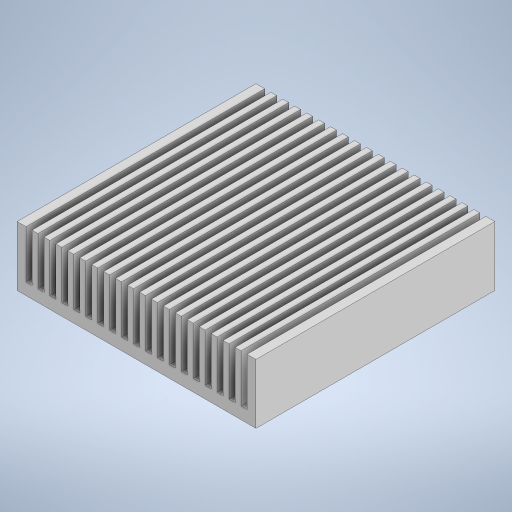
# Autodesk Inventor part: cooling_fin
Saved by Autodesk Inventor 2023 (Build 270158000, 158)
## iProperties
Created: 2023-07-12
Part Number: cooling_fin
Material: 一般
Document SubType Name: Modeling
Designer: 310611102
Density: 1 g/cm^3
Appearance: 預設
Author: 310611102
Autodesk Inventor part; units mm, degrees
ref_plane "YZ Plane" through (0, 0, 0) normal (1, 0, 0) x (0, 1, 0)
ref_plane "XZ Plane" through (0, 0, 0) normal (0, 1, 0) x (-1, 0, 0)
ref_plane "XY Plane" through (0, 0, 0) normal (0, 0, 1) x (1, 0, 0)
sketch "Sketch1" plane through (0, 0, 0) normal (0, 0, 1) x (1, 0, 0)
  line L0 (-10, 2.5) -> (10, 2.5)
  line L1 (10, 2.5) -> (10, -2.5)
  line L2 (10, -2.5) -> (-10, -2.5)
  line L3 (-10, -2.5) -> (-10, 2.5)
  line L4 (-10, 2.5) -> (10, -2.5) construction
  line L5 (10, 2.5) -> (-10, -2.5) construction
  point P0 (0, 0)
  dimension "d0" = 20
  dimension "d1" = 5
  constraints: 12 end point, 2 midpoint, 2 parallel, 1 horizontal, 1 perpendicular
  measures "d0" distance of L0.start L0.end
  measures "d1" distance of L0.end L1.end
extrude "Extrusion1" add sketch "Sketch1" along normal blind 20
sketch "Sketch2" plane through (0, 0, 20) normal (0, 0, 1) x (1, 0, 0)
  line L0 (-0.25, 3.3824) -> (0.25, 3.3824)
  line L1 (0.25, 3.3824) -> (0.25, -1.5)
  line L2 (0.25, -1.5) -> (-0.25, -1.5)
  line L3 (-0.25, -1.5) -> (-0.25, 3.3824)
  line L4 (-0.25, 3.3824) -> (0.25, -1.5) construction
  line L5 (0.25, 3.3824) -> (-0.25, -1.5) construction
  line L6 (-10, -2.5) -> (10, -2.5) projected
  line L7 (0.75, 3.3824) -> (1.25, 3.3824)
  line L8 (1.25, 3.3824) -> (1.25, -1.5)
  line L9 (1.25, -1.5) -> (0.75, -1.5)
  line L10 (0.75, -1.5) -> (0.75, 3.3824)
  line L11 (0.75, 3.3824) -> (1.25, -1.5) construction
  line L12 (1.25, 3.3824) -> (0.75, -1.5) construction
  line L13 (1.75, 3.3824) -> (2.25, 3.3824)
  line L14 (2.25, 3.3824) -> (2.25, -1.5)
  line L15 (2.25, -1.5) -> (1.75, -1.5)
  line L16 (1.75, -1.5) -> (1.75, 3.3824)
  line L17 (1.75, 3.3824) -> (2.25, -1.5) construction
  line L18 (2.25, 3.3824) -> (1.75, -1.5) construction
  line L19 (2.75, 3.3824) -> (3.25, 3.3824)
  line L20 (3.25, 3.3824) -> (3.25, -1.5)
  line L21 (3.25, -1.5) -> (2.75, -1.5)
  line L22 (2.75, -1.5) -> (2.75, 3.3824)
  line L23 (2.75, 3.3824) -> (3.25, -1.5) construction
  line L24 (3.25, 3.3824) -> (2.75, -1.5) construction
  line L25 (3.75, 3.3824) -> (4.25, 3.3824)
  line L26 (4.25, 3.3824) -> (4.25, -1.5)
  line L27 (4.25, -1.5) -> (3.75, -1.5)
  line L28 (3.75, -1.5) -> (3.75, 3.3824)
  line L29 (3.75, 3.3824) -> (4.25, -1.5) construction
  line L30 (4.25, 3.3824) -> (3.75, -1.5) construction
  line L31 (4.75, 3.3824) -> (5.25, 3.3824)
  line L32 (5.25, 3.3824) -> (5.25, -1.5)
  line L33 (5.25, -1.5) -> (4.75, -1.5)
  line L34 (4.75, -1.5) -> (4.75, 3.3824)
  line L35 (4.75, 3.3824) -> (5.25, -1.5) construction
  line L36 (5.25, 3.3824) -> (4.75, -1.5) construction
  line L37 (5.75, 3.3824) -> (6.25, 3.3824)
  line L38 (6.25, 3.3824) -> (6.25, -1.5)
  line L39 (6.25, -1.5) -> (5.75, -1.5)
  line L40 (5.75, -1.5) -> (5.75, 3.3824)
  line L41 (5.75, 3.3824) -> (6.25, -1.5) construction
  line L42 (6.25, 3.3824) -> (5.75, -1.5) construction
  line L43 (6.75, 3.3824) -> (7.25, 3.3824)
  line L44 (7.25, 3.3824) -> (7.25, -1.5)
  line L45 (7.25, -1.5) -> (6.75, -1.5)
  line L46 (6.75, -1.5) -> (6.75, 3.3824)
  line L47 (6.75, 3.3824) -> (7.25, -1.5) construction
  line L48 (7.25, 3.3824) -> (6.75, -1.5) construction
  line L49 (7.75, 3.3824) -> (8.25, 3.3824)
  line L50 (8.25, 3.3824) -> (8.25, -1.5)
  line L51 (8.25, -1.5) -> (7.75, -1.5)
  line L52 (7.75, -1.5) -> (7.75, 3.3824)
  line L53 (7.75, 3.3824) -> (8.25, -1.5) construction
  line L54 (8.25, 3.3824) -> (7.75, -1.5) construction
  line L55 (8.75, 3.3824) -> (9.25, 3.3824)
  line L56 (9.25, 3.3824) -> (9.25, -1.5)
  line L57 (9.25, -1.5) -> (8.75, -1.5)
  line L58 (8.75, -1.5) -> (8.75, 3.3824)
  line L59 (8.75, 3.3824) -> (9.25, -1.5) construction
  line L60 (9.25, 3.3824) -> (8.75, -1.5) construction
  line L61 (-1.25, 3.3824) -> (-0.75, 3.3824)
  line L62 (-0.75, 3.3824) -> (-0.75, -1.5)
  line L63 (-0.75, -1.5) -> (-1.25, -1.5)
  line L64 (-1.25, -1.5) -> (-1.25, 3.3824)
  line L65 (-1.25, 3.3824) -> (-0.75, -1.5) construction
  line L66 (-0.75, 3.3824) -> (-1.25, -1.5) construction
  line L67 (-0.25, 3.3824) -> (0.25, 3.3824)
  line L68 (0.25, 3.3824) -> (0.25, -1.5)
  line L69 (0.25, -1.5) -> (-0.25, -1.5)
  line L70 (-0.25, -1.5) -> (-0.25, 3.3824)
  line L71 (-0.25, 3.3824) -> (0.25, -1.5) construction
  line L72 (0.25, 3.3824) -> (-0.25, -1.5) construction
  line L73 (0.75, 3.3824) -> (1.25, 3.3824)
  line L74 (1.25, 3.3824) -> (1.25, -1.5)
  line L75 (1.25, -1.5) -> (0.75, -1.5)
  line L76 (0.75, -1.5) -> (0.75, 3.3824)
  line L77 (0.75, 3.3824) -> (1.25, -1.5) construction
  line L78 (1.25, 3.3824) -> (0.75, -1.5) construction
  line L79 (1.75, 3.3824) -> (2.25, 3.3824)
  line L80 (2.25, 3.3824) -> (2.25, -1.5)
  line L81 (2.25, -1.5) -> (1.75, -1.5)
  line L82 (1.75, -1.5) -> (1.75, 3.3824)
  line L83 (1.75, 3.3824) -> (2.25, -1.5) construction
  line L84 (2.25, 3.3824) -> (1.75, -1.5) construction
  line L85 (2.75, 3.3824) -> (3.25, 3.3824)
  line L86 (3.25, 3.3824) -> (3.25, -1.5)
  line L87 (3.25, -1.5) -> (2.75, -1.5)
  line L88 (2.75, -1.5) -> (2.75, 3.3824)
  line L89 (2.75, 3.3824) -> (3.25, -1.5) construction
  line L90 (3.25, 3.3824) -> (2.75, -1.5) construction
  line L91 (3.75, 3.3824) -> (4.25, 3.3824)
  line L92 (4.25, 3.3824) -> (4.25, -1.5)
  line L93 (4.25, -1.5) -> (3.75, -1.5)
  line L94 (3.75, -1.5) -> (3.75, 3.3824)
  line L95 (3.75, 3.3824) -> (4.25, -1.5) construction
  line L96 (4.25, 3.3824) -> (3.75, -1.5) construction
  line L97 (4.75, 3.3824) -> (5.25, 3.3824)
  line L98 (5.25, 3.3824) -> (5.25, -1.5)
  line L99 (5.25, -1.5) -> (4.75, -1.5)
  line L100 (4.75, -1.5) -> (4.75, 3.3824)
  line L101 (4.75, 3.3824) -> (5.25, -1.5) construction
  line L102 (5.25, 3.3824) -> (4.75, -1.5) construction
  line L103 (5.75, 3.3824) -> (6.25, 3.3824)
  line L104 (6.25, 3.3824) -> (6.25, -1.5)
  line L105 (6.25, -1.5) -> (5.75, -1.5)
  line L106 (5.75, -1.5) -> (5.75, 3.3824)
  line L107 (5.75, 3.3824) -> (6.25, -1.5) construction
  line L108 (6.25, 3.3824) -> (5.75, -1.5) construction
  line L109 (6.75, 3.3824) -> (7.25, 3.3824)
  line L110 (7.25, 3.3824) -> (7.25, -1.5)
  line L111 (7.25, -1.5) -> (6.75, -1.5)
  line L112 (6.75, -1.5) -> (6.75, 3.3824)
  line L113 (6.75, 3.3824) -> (7.25, -1.5) construction
  line L114 (7.25, 3.3824) -> (6.75, -1.5) construction
  line L115 (7.75, 3.3824) -> (8.25, 3.3824)
  line L116 (8.25, 3.3824) -> (8.25, -1.5)
  line L117 (8.25, -1.5) -> (7.75, -1.5)
  line L118 (7.75, -1.5) -> (7.75, 3.3824)
  line L119 (7.75, 3.3824) -> (8.25, -1.5) construction
  line L120 (8.25, 3.3824) -> (7.75, -1.5) construction
  line L121 (-2.25, 3.3824) -> (-1.75, 3.3824)
  line L122 (-1.75, 3.3824) -> (-1.75, -1.5)
  line L123 (-1.75, -1.5) -> (-2.25, -1.5)
  line L124 (-2.25, -1.5) -> (-2.25, 3.3824)
  line L125 (-2.25, 3.3824) -> (-1.75, -1.5) construction
  line L126 (-1.75, 3.3824) -> (-2.25, -1.5) construction
  line L127 (-1.25, 3.3824) -> (-0.75, 3.3824)
  line L128 (-0.75, 3.3824) -> (-0.75, -1.5)
  line L129 (-0.75, -1.5) -> (-1.25, -1.5)
  line L130 (-1.25, -1.5) -> (-1.25, 3.3824)
  line L131 (-1.25, 3.3824) -> (-0.75, -1.5) construction
  line L132 (-0.75, 3.3824) -> (-1.25, -1.5) construction
  line L133 (-0.25, 3.3824) -> (0.25, 3.3824)
  line L134 (0.25, 3.3824) -> (0.25, -1.5)
  line L135 (0.25, -1.5) -> (-0.25, -1.5)
  line L136 (-0.25, -1.5) -> (-0.25, 3.3824)
  line L137 (-0.25, 3.3824) -> (0.25, -1.5) construction
  line L138 (0.25, 3.3824) -> (-0.25, -1.5) construction
  line L139 (0.75, 3.3824) -> (1.25, 3.3824)
  line L140 (1.25, 3.3824) -> (1.25, -1.5)
  line L141 (1.25, -1.5) -> (0.75, -1.5)
  line L142 (0.75, -1.5) -> (0.75, 3.3824)
  line L143 (0.75, 3.3824) -> (1.25, -1.5) construction
  line L144 (1.25, 3.3824) -> (0.75, -1.5) construction
  line L145 (1.75, 3.3824) -> (2.25, 3.3824)
  line L146 (2.25, 3.3824) -> (2.25, -1.5)
  line L147 (2.25, -1.5) -> (1.75, -1.5)
  line L148 (1.75, -1.5) -> (1.75, 3.3824)
  line L149 (1.75, 3.3824) -> (2.25, -1.5) construction
  line L150 (2.25, 3.3824) -> (1.75, -1.5) construction
  line L151 (2.75, 3.3824) -> (3.25, 3.3824)
  line L152 (3.25, 3.3824) -> (3.25, -1.5)
  line L153 (3.25, -1.5) -> (2.75, -1.5)
  line L154 (2.75, -1.5) -> (2.75, 3.3824)
  line L155 (2.75, 3.3824) -> (3.25, -1.5) construction
  line L156 (3.25, 3.3824) -> (2.75, -1.5) construction
  line L157 (3.75, 3.3824) -> (4.25, 3.3824)
  line L158 (4.25, 3.3824) -> (4.25, -1.5)
  line L159 (4.25, -1.5) -> (3.75, -1.5)
  line L160 (3.75, -1.5) -> (3.75, 3.3824)
  line L161 (3.75, 3.3824) -> (4.25, -1.5) construction
  line L162 (4.25, 3.3824) -> (3.75, -1.5) construction
  line L163 (4.75, 3.3824) -> (5.25, 3.3824)
  line L164 (5.25, 3.3824) -> (5.25, -1.5)
  line L165 (5.25, -1.5) -> (4.75, -1.5)
  line L166 (4.75, -1.5) -> (4.75, 3.3824)
  line L167 (4.75, 3.3824) -> (5.25, -1.5) construction
  line L168 (5.25, 3.3824) -> (4.75, -1.5) construction
  line L169 (5.75, 3.3824) -> (6.25, 3.3824)
  line L170 (6.25, 3.3824) -> (6.25, -1.5)
  line L171 (6.25, -1.5) -> (5.75, -1.5)
  line L172 (5.75, -1.5) -> (5.75, 3.3824)
  line L173 (5.75, 3.3824) -> (6.25, -1.5) construction
  line L174 (6.25, 3.3824) -> (5.75, -1.5) construction
  line L175 (6.75, 3.3824) -> (7.25, 3.3824)
  line L176 (7.25, 3.3824) -> (7.25, -1.5)
  line L177 (7.25, -1.5) -> (6.75, -1.5)
  line L178 (6.75, -1.5) -> (6.75, 3.3824)
  line L179 (6.75, 3.3824) -> (7.25, -1.5) construction
  line L180 (7.25, 3.3824) -> (6.75, -1.5) construction
  line L181 (-3.25, 3.3824) -> (-2.75, 3.3824)
  line L182 (-2.75, 3.3824) -> (-2.75, -1.5)
  line L183 (-2.75, -1.5) -> (-3.25, -1.5)
  line L184 (-3.25, -1.5) -> (-3.25, 3.3824)
  line L185 (-3.25, 3.3824) -> (-2.75, -1.5) construction
  line L186 (-2.75, 3.3824) -> (-3.25, -1.5) construction
  line L187 (-2.25, 3.3824) -> (-1.75, 3.3824)
  line L188 (-1.75, 3.3824) -> (-1.75, -1.5)
  line L189 (-1.75, -1.5) -> (-2.25, -1.5)
  line L190 (-2.25, -1.5) -> (-2.25, 3.3824)
  line L191 (-2.25, 3.3824) -> (-1.75, -1.5) construction
  line L192 (-1.75, 3.3824) -> (-2.25, -1.5) construction
  line L193 (-1.25, 3.3824) -> (-0.75, 3.3824)
  line L194 (-0.75, 3.3824) -> (-0.75, -1.5)
  line L195 (-0.75, -1.5) -> (-1.25, -1.5)
  line L196 (-1.25, -1.5) -> (-1.25, 3.3824)
  line L197 (-1.25, 3.3824) -> (-0.75, -1.5) construction
  line L198 (-0.75, 3.3824) -> (-1.25, -1.5) construction
  line L199 (-0.25, 3.3824) -> (0.25, 3.3824)
  line L200 (0.25, 3.3824) -> (0.25, -1.5)
  line L201 (0.25, -1.5) -> (-0.25, -1.5)
  line L202 (-0.25, -1.5) -> (-0.25, 3.3824)
  line L203 (-0.25, 3.3824) -> (0.25, -1.5) construction
  line L204 (0.25, 3.3824) -> (-0.25, -1.5) construction
  line L205 (0.75, 3.3824) -> (1.25, 3.3824)
  line L206 (1.25, 3.3824) -> (1.25, -1.5)
  line L207 (1.25, -1.5) -> (0.75, -1.5)
  line L208 (0.75, -1.5) -> (0.75, 3.3824)
  line L209 (0.75, 3.3824) -> (1.25, -1.5) construction
  line L210 (1.25, 3.3824) -> (0.75, -1.5) construction
  line L211 (1.75, 3.3824) -> (2.25, 3.3824)
  line L212 (2.25, 3.3824) -> (2.25, -1.5)
  line L213 (2.25, -1.5) -> (1.75, -1.5)
  line L214 (1.75, -1.5) -> (1.75, 3.3824)
  line L215 (1.75, 3.3824) -> (2.25, -1.5) construction
  line L216 (2.25, 3.3824) -> (1.75, -1.5) construction
  line L217 (2.75, 3.3824) -> (3.25, 3.3824)
  line L218 (3.25, 3.3824) -> (3.25, -1.5)
  line L219 (3.25, -1.5) -> (2.75, -1.5)
  line L220 (2.75, -1.5) -> (2.75, 3.3824)
  line L221 (2.75, 3.3824) -> (3.25, -1.5) construction
  line L222 (3.25, 3.3824) -> (2.75, -1.5) construction
  line L223 (3.75, 3.3824) -> (4.25, 3.3824)
  line L224 (4.25, 3.3824) -> (4.25, -1.5)
  line L225 (4.25, -1.5) -> (3.75, -1.5)
  line L226 (3.75, -1.5) -> (3.75, 3.3824)
  line L227 (3.75, 3.3824) -> (4.25, -1.5) construction
  line L228 (4.25, 3.3824) -> (3.75, -1.5) construction
  line L229 (4.75, 3.3824) -> (5.25, 3.3824)
  line L230 (5.25, 3.3824) -> (5.25, -1.5)
  line L231 (5.25, -1.5) -> (4.75, -1.5)
  line L232 (4.75, -1.5) -> (4.75, 3.3824)
  line L233 (4.75, 3.3824) -> (5.25, -1.5) construction
  line L234 (5.25, 3.3824) -> (4.75, -1.5) construction
  line L235 (5.75, 3.3824) -> (6.25, 3.3824)
  line L236 (6.25, 3.3824) -> (6.25, -1.5)
  line L237 (6.25, -1.5) -> (5.75, -1.5)
  line L238 (5.75, -1.5) -> (5.75, 3.3824)
  line L239 (5.75, 3.3824) -> (6.25, -1.5) construction
  line L240 (6.25, 3.3824) -> (5.75, -1.5) construction
  line L241 (-4.25, 3.3824) -> (-3.75, 3.3824)
  line L242 (-3.75, 3.3824) -> (-3.75, -1.5)
  line L243 (-3.75, -1.5) -> (-4.25, -1.5)
  line L244 (-4.25, -1.5) -> (-4.25, 3.3824)
  line L245 (-4.25, 3.3824) -> (-3.75, -1.5) construction
  line L246 (-3.75, 3.3824) -> (-4.25, -1.5) construction
  line L247 (-3.25, 3.3824) -> (-2.75, 3.3824)
  line L248 (-2.75, 3.3824) -> (-2.75, -1.5)
  line L249 (-2.75, -1.5) -> (-3.25, -1.5)
  line L250 (-3.25, -1.5) -> (-3.25, 3.3824)
  line L251 (-3.25, 3.3824) -> (-2.75, -1.5) construction
  line L252 (-2.75, 3.3824) -> (-3.25, -1.5) construction
  line L253 (-2.25, 3.3824) -> (-1.75, 3.3824)
  line L254 (-1.75, 3.3824) -> (-1.75, -1.5)
  line L255 (-1.75, -1.5) -> (-2.25, -1.5)
  line L256 (-2.25, -1.5) -> (-2.25, 3.3824)
  line L257 (-2.25, 3.3824) -> (-1.75, -1.5) construction
  line L258 (-1.75, 3.3824) -> (-2.25, -1.5) construction
  line L259 (-1.25, 3.3824) -> (-0.75, 3.3824)
  line L260 (-0.75, 3.3824) -> (-0.75, -1.5)
  line L261 (-0.75, -1.5) -> (-1.25, -1.5)
  line L262 (-1.25, -1.5) -> (-1.25, 3.3824)
  line L263 (-1.25, 3.3824) -> (-0.75, -1.5) construction
  line L264 (-0.75, 3.3824) -> (-1.25, -1.5) construction
  line L265 (-0.25, 3.3824) -> (0.25, 3.3824)
  line L266 (0.25, 3.3824) -> (0.25, -1.5)
  line L267 (0.25, -1.5) -> (-0.25, -1.5)
  line L268 (-0.25, -1.5) -> (-0.25, 3.3824)
  line L269 (-0.25, 3.3824) -> (0.25, -1.5) construction
  line L270 (0.25, 3.3824) -> (-0.25, -1.5) construction
  line L271 (0.75, 3.3824) -> (1.25, 3.3824)
  line L272 (1.25, 3.3824) -> (1.25, -1.5)
  line L273 (1.25, -1.5) -> (0.75, -1.5)
  line L274 (0.75, -1.5) -> (0.75, 3.3824)
  line L275 (0.75, 3.3824) -> (1.25, -1.5) construction
  line L276 (1.25, 3.3824) -> (0.75, -1.5) construction
  line L277 (1.75, 3.3824) -> (2.25, 3.3824)
  line L278 (2.25, 3.3824) -> (2.25, -1.5)
  line L279 (2.25, -1.5) -> (1.75, -1.5)
  line L280 (1.75, -1.5) -> (1.75, 3.3824)
  line L281 (1.75, 3.3824) -> (2.25, -1.5) construction
  line L282 (2.25, 3.3824) -> (1.75, -1.5) construction
  line L283 (2.75, 3.3824) -> (3.25, 3.3824)
  line L284 (3.25, 3.3824) -> (3.25, -1.5)
  line L285 (3.25, -1.5) -> (2.75, -1.5)
  line L286 (2.75, -1.5) -> (2.75, 3.3824)
  line L287 (2.75, 3.3824) -> (3.25, -1.5) construction
  line L288 (3.25, 3.3824) -> (2.75, -1.5) construction
  line L289 (3.75, 3.3824) -> (4.25, 3.3824)
  line L290 (4.25, 3.3824) -> (4.25, -1.5)
  line L291 (4.25, -1.5) -> (3.75, -1.5)
  line L292 (3.75, -1.5) -> (3.75, 3.3824)
  line L293 (3.75, 3.3824) -> (4.25, -1.5) construction
  line L294 (4.25, 3.3824) -> (3.75, -1.5) construction
  line L295 (4.75, 3.3824) -> (5.25, 3.3824)
  line L296 (5.25, 3.3824) -> (5.25, -1.5)
  line L297 (5.25, -1.5) -> (4.75, -1.5)
  line L298 (4.75, -1.5) -> (4.75, 3.3824)
  line L299 (4.75, 3.3824) -> (5.25, -1.5) construction
  line L300 (5.25, 3.3824) -> (4.75, -1.5) construction
  line L301 (-5.25, 3.3824) -> (-4.75, 3.3824)
  line L302 (-4.75, 3.3824) -> (-4.75, -1.5)
  line L303 (-4.75, -1.5) -> (-5.25, -1.5)
  line L304 (-5.25, -1.5) -> (-5.25, 3.3824)
  line L305 (-5.25, 3.3824) -> (-4.75, -1.5) construction
  line L306 (-4.75, 3.3824) -> (-5.25, -1.5) construction
  line L307 (-4.25, 3.3824) -> (-3.75, 3.3824)
  line L308 (-3.75, 3.3824) -> (-3.75, -1.5)
  line L309 (-3.75, -1.5) -> (-4.25, -1.5)
  line L310 (-4.25, -1.5) -> (-4.25, 3.3824)
  line L311 (-4.25, 3.3824) -> (-3.75, -1.5) construction
  line L312 (-3.75, 3.3824) -> (-4.25, -1.5) construction
  line L313 (-3.25, 3.3824) -> (-2.75, 3.3824)
  line L314 (-2.75, 3.3824) -> (-2.75, -1.5)
  line L315 (-2.75, -1.5) -> (-3.25, -1.5)
  line L316 (-3.25, -1.5) -> (-3.25, 3.3824)
  line L317 (-3.25, 3.3824) -> (-2.75, -1.5) construction
  line L318 (-2.75, 3.3824) -> (-3.25, -1.5) construction
  line L319 (-2.25, 3.3824) -> (-1.75, 3.3824)
  line L320 (-1.75, 3.3824) -> (-1.75, -1.5)
  line L321 (-1.75, -1.5) -> (-2.25, -1.5)
  line L322 (-2.25, -1.5) -> (-2.25, 3.3824)
  line L323 (-2.25, 3.3824) -> (-1.75, -1.5) construction
  line L324 (-1.75, 3.3824) -> (-2.25, -1.5) construction
  line L325 (-1.25, 3.3824) -> (-0.75, 3.3824)
  line L326 (-0.75, 3.3824) -> (-0.75, -1.5)
  line L327 (-0.75, -1.5) -> (-1.25, -1.5)
  line L328 (-1.25, -1.5) -> (-1.25, 3.3824)
  line L329 (-1.25, 3.3824) -> (-0.75, -1.5) construction
  line L330 (-0.75, 3.3824) -> (-1.25, -1.5) construction
  line L331 (-0.25, 3.3824) -> (0.25, 3.3824)
  line L332 (0.25, 3.3824) -> (0.25, -1.5)
  line L333 (0.25, -1.5) -> (-0.25, -1.5)
  line L334 (-0.25, -1.5) -> (-0.25, 3.3824)
  line L335 (-0.25, 3.3824) -> (0.25, -1.5) construction
  line L336 (0.25, 3.3824) -> (-0.25, -1.5) construction
  line L337 (0.75, 3.3824) -> (1.25, 3.3824)
  line L338 (1.25, 3.3824) -> (1.25, -1.5)
  line L339 (1.25, -1.5) -> (0.75, -1.5)
  line L340 (0.75, -1.5) -> (0.75, 3.3824)
  line L341 (0.75, 3.3824) -> (1.25, -1.5) construction
  line L342 (1.25, 3.3824) -> (0.75, -1.5) construction
  line L343 (1.75, 3.3824) -> (2.25, 3.3824)
  line L344 (2.25, 3.3824) -> (2.25, -1.5)
  line L345 (2.25, -1.5) -> (1.75, -1.5)
  line L346 (1.75, -1.5) -> (1.75, 3.3824)
  line L347 (1.75, 3.3824) -> (2.25, -1.5) construction
  line L348 (2.25, 3.3824) -> (1.75, -1.5) construction
  line L349 (2.75, 3.3824) -> (3.25, 3.3824)
  line L350 (3.25, 3.3824) -> (3.25, -1.5)
  line L351 (3.25, -1.5) -> (2.75, -1.5)
  line L352 (2.75, -1.5) -> (2.75, 3.3824)
  line L353 (2.75, 3.3824) -> (3.25, -1.5) construction
  line L354 (3.25, 3.3824) -> (2.75, -1.5) construction
  line L355 (3.75, 3.3824) -> (4.25, 3.3824)
  line L356 (4.25, 3.3824) -> (4.25, -1.5)
  line L357 (4.25, -1.5) -> (3.75, -1.5)
  line L358 (3.75, -1.5) -> (3.75, 3.3824)
  line L359 (3.75, 3.3824) -> (4.25, -1.5) construction
  line L360 (4.25, 3.3824) -> (3.75, -1.5) construction
  line L361 (-6.25, 3.3824) -> (-5.75, 3.3824)
  line L362 (-5.75, 3.3824) -> (-5.75, -1.5)
  line L363 (-5.75, -1.5) -> (-6.25, -1.5)
  line L364 (-6.25, -1.5) -> (-6.25, 3.3824)
  line L365 (-6.25, 3.3824) -> (-5.75, -1.5) construction
  line L366 (-5.75, 3.3824) -> (-6.25, -1.5) construction
  line L367 (-5.25, 3.3824) -> (-4.75, 3.3824)
  line L368 (-4.75, 3.3824) -> (-4.75, -1.5)
  line L369 (-4.75, -1.5) -> (-5.25, -1.5)
  line L370 (-5.25, -1.5) -> (-5.25, 3.3824)
  line L371 (-5.25, 3.3824) -> (-4.75, -1.5) construction
  line L372 (-4.75, 3.3824) -> (-5.25, -1.5) construction
  line L373 (-4.25, 3.3824) -> (-3.75, 3.3824)
  line L374 (-3.75, 3.3824) -> (-3.75, -1.5)
  line L375 (-3.75, -1.5) -> (-4.25, -1.5)
  line L376 (-4.25, -1.5) -> (-4.25, 3.3824)
  line L377 (-4.25, 3.3824) -> (-3.75, -1.5) construction
  line L378 (-3.75, 3.3824) -> (-4.25, -1.5) construction
  line L379 (-3.25, 3.3824) -> (-2.75, 3.3824)
  line L380 (-2.75, 3.3824) -> (-2.75, -1.5)
  line L381 (-2.75, -1.5) -> (-3.25, -1.5)
  line L382 (-3.25, -1.5) -> (-3.25, 3.3824)
  line L383 (-3.25, 3.3824) -> (-2.75, -1.5) construction
  line L384 (-2.75, 3.3824) -> (-3.25, -1.5) construction
  line L385 (-2.25, 3.3824) -> (-1.75, 3.3824)
  line L386 (-1.75, 3.3824) -> (-1.75, -1.5)
  line L387 (-1.75, -1.5) -> (-2.25, -1.5)
  line L388 (-2.25, -1.5) -> (-2.25, 3.3824)
  line L389 (-2.25, 3.3824) -> (-1.75, -1.5) construction
  line L390 (-1.75, 3.3824) -> (-2.25, -1.5) construction
  line L391 (-1.25, 3.3824) -> (-0.75, 3.3824)
  line L392 (-0.75, 3.3824) -> (-0.75, -1.5)
  line L393 (-0.75, -1.5) -> (-1.25, -1.5)
  line L394 (-1.25, -1.5) -> (-1.25, 3.3824)
  line L395 (-1.25, 3.3824) -> (-0.75, -1.5) construction
  line L396 (-0.75, 3.3824) -> (-1.25, -1.5) construction
  line L397 (-0.25, 3.3824) -> (0.25, 3.3824)
  line L398 (0.25, 3.3824) -> (0.25, -1.5)
  line L399 (0.25, -1.5) -> (-0.25, -1.5)
  line L400 (-0.25, -1.5) -> (-0.25, 3.3824)
  line L401 (-0.25, 3.3824) -> (0.25, -1.5) construction
  line L402 (0.25, 3.3824) -> (-0.25, -1.5) construction
  line L403 (0.75, 3.3824) -> (1.25, 3.3824)
  line L404 (1.25, 3.3824) -> (1.25, -1.5)
  line L405 (1.25, -1.5) -> (0.75, -1.5)
  line L406 (0.75, -1.5) -> (0.75, 3.3824)
  line L407 (0.75, 3.3824) -> (1.25, -1.5) construction
  line L408 (1.25, 3.3824) -> (0.75, -1.5) construction
  line L409 (1.75, 3.3824) -> (2.25, 3.3824)
  line L410 (2.25, 3.3824) -> (2.25, -1.5)
  line L411 (2.25, -1.5) -> (1.75, -1.5)
  line L412 (1.75, -1.5) -> (1.75, 3.3824)
  line L413 (1.75, 3.3824) -> (2.25, -1.5) construction
  line L414 (2.25, 3.3824) -> (1.75, -1.5) construction
  line L415 (2.75, 3.3824) -> (3.25, 3.3824)
  line L416 (3.25, 3.3824) -> (3.25, -1.5)
  line L417 (3.25, -1.5) -> (2.75, -1.5)
  line L418 (2.75, -1.5) -> (2.75, 3.3824)
  line L419 (2.75, 3.3824) -> (3.25, -1.5) construction
  line L420 (3.25, 3.3824) -> (2.75, -1.5) construction
  line L421 (-7.25, 3.3824) -> (-6.75, 3.3824)
  line L422 (-6.75, 3.3824) -> (-6.75, -1.5)
  line L423 (-6.75, -1.5) -> (-7.25, -1.5)
  line L424 (-7.25, -1.5) -> (-7.25, 3.3824)
  line L425 (-7.25, 3.3824) -> (-6.75, -1.5) construction
  line L426 (-6.75, 3.3824) -> (-7.25, -1.5) construction
  line L427 (-6.25, 3.3824) -> (-5.75, 3.3824)
  line L428 (-5.75, 3.3824) -> (-5.75, -1.5)
  line L429 (-5.75, -1.5) -> (-6.25, -1.5)
  line L430 (-6.25, -1.5) -> (-6.25, 3.3824)
  line L431 (-6.25, 3.3824) -> (-5.75, -1.5) construction
  line L432 (-5.75, 3.3824) -> (-6.25, -1.5) construction
  line L433 (-5.25, 3.3824) -> (-4.75, 3.3824)
  line L434 (-4.75, 3.3824) -> (-4.75, -1.5)
  line L435 (-4.75, -1.5) -> (-5.25, -1.5)
  line L436 (-5.25, -1.5) -> (-5.25, 3.3824)
  line L437 (-5.25, 3.3824) -> (-4.75, -1.5) construction
  line L438 (-4.75, 3.3824) -> (-5.25, -1.5) construction
  line L439 (-4.25, 3.3824) -> (-3.75, 3.3824)
  line L440 (-3.75, 3.3824) -> (-3.75, -1.5)
  line L441 (-3.75, -1.5) -> (-4.25, -1.5)
  line L442 (-4.25, -1.5) -> (-4.25, 3.3824)
  line L443 (-4.25, 3.3824) -> (-3.75, -1.5) construction
  line L444 (-3.75, 3.3824) -> (-4.25, -1.5) construction
  line L445 (-3.25, 3.3824) -> (-2.75, 3.3824)
  line L446 (-2.75, 3.3824) -> (-2.75, -1.5)
  line L447 (-2.75, -1.5) -> (-3.25, -1.5)
  line L448 (-3.25, -1.5) -> (-3.25, 3.3824)
  line L449 (-3.25, 3.3824) -> (-2.75, -1.5) construction
  line L450 (-2.75, 3.3824) -> (-3.25, -1.5) construction
  line L451 (-2.25, 3.3824) -> (-1.75, 3.3824)
  line L452 (-1.75, 3.3824) -> (-1.75, -1.5)
  line L453 (-1.75, -1.5) -> (-2.25, -1.5)
  line L454 (-2.25, -1.5) -> (-2.25, 3.3824)
  line L455 (-2.25, 3.3824) -> (-1.75, -1.5) construction
  line L456 (-1.75, 3.3824) -> (-2.25, -1.5) construction
  line L457 (-1.25, 3.3824) -> (-0.75, 3.3824)
  line L458 (-0.75, 3.3824) -> (-0.75, -1.5)
  line L459 (-0.75, -1.5) -> (-1.25, -1.5)
  line L460 (-1.25, -1.5) -> (-1.25, 3.3824)
  line L461 (-1.25, 3.3824) -> (-0.75, -1.5) construction
  line L462 (-0.75, 3.3824) -> (-1.25, -1.5) construction
  line L463 (-0.25, 3.3824) -> (0.25, 3.3824)
  line L464 (0.25, 3.3824) -> (0.25, -1.5)
  line L465 (0.25, -1.5) -> (-0.25, -1.5)
  line L466 (-0.25, -1.5) -> (-0.25, 3.3824)
  line L467 (-0.25, 3.3824) -> (0.25, -1.5) construction
  line L468 (0.25, 3.3824) -> (-0.25, -1.5) construction
  line L469 (0.75, 3.3824) -> (1.25, 3.3824)
  line L470 (1.25, 3.3824) -> (1.25, -1.5)
  line L471 (1.25, -1.5) -> (0.75, -1.5)
  line L472 (0.75, -1.5) -> (0.75, 3.3824)
  line L473 (0.75, 3.3824) -> (1.25, -1.5) construction
  line L474 (1.25, 3.3824) -> (0.75, -1.5) construction
  line L475 (1.75, 3.3824) -> (2.25, 3.3824)
  line L476 (2.25, 3.3824) -> (2.25, -1.5)
  line L477 (2.25, -1.5) -> (1.75, -1.5)
  line L478 (1.75, -1.5) -> (1.75, 3.3824)
  line L479 (1.75, 3.3824) -> (2.25, -1.5) construction
  line L480 (2.25, 3.3824) -> (1.75, -1.5) construction
  line L481 (-8.25, 3.3824) -> (-7.75, 3.3824)
  line L482 (-7.75, 3.3824) -> (-7.75, -1.5)
  line L483 (-7.75, -1.5) -> (-8.25, -1.5)
  line L484 (-8.25, -1.5) -> (-8.25, 3.3824)
  line L485 (-8.25, 3.3824) -> (-7.75, -1.5) construction
  line L486 (-7.75, 3.3824) -> (-8.25, -1.5) construction
  line L487 (-7.25, 3.3824) -> (-6.75, 3.3824)
  line L488 (-6.75, 3.3824) -> (-6.75, -1.5)
  line L489 (-6.75, -1.5) -> (-7.25, -1.5)
  line L490 (-7.25, -1.5) -> (-7.25, 3.3824)
  line L491 (-7.25, 3.3824) -> (-6.75, -1.5) construction
  line L492 (-6.75, 3.3824) -> (-7.25, -1.5) construction
  line L493 (-6.25, 3.3824) -> (-5.75, 3.3824)
  line L494 (-5.75, 3.3824) -> (-5.75, -1.5)
  line L495 (-5.75, -1.5) -> (-6.25, -1.5)
  line L496 (-6.25, -1.5) -> (-6.25, 3.3824)
  line L497 (-6.25, 3.3824) -> (-5.75, -1.5) construction
  line L498 (-5.75, 3.3824) -> (-6.25, -1.5) construction
  line L499 (-5.25, 3.3824) -> (-4.75, 3.3824)
  line L500 (-4.75, 3.3824) -> (-4.75, -1.5)
  line L501 (-4.75, -1.5) -> (-5.25, -1.5)
  line L502 (-5.25, -1.5) -> (-5.25, 3.3824)
  line L503 (-5.25, 3.3824) -> (-4.75, -1.5) construction
  line L504 (-4.75, 3.3824) -> (-5.25, -1.5) construction
  line L505 (-4.25, 3.3824) -> (-3.75, 3.3824)
  line L506 (-3.75, 3.3824) -> (-3.75, -1.5)
  line L507 (-3.75, -1.5) -> (-4.25, -1.5)
  line L508 (-4.25, -1.5) -> (-4.25, 3.3824)
  line L509 (-4.25, 3.3824) -> (-3.75, -1.5) construction
  line L510 (-3.75, 3.3824) -> (-4.25, -1.5) construction
  line L511 (-3.25, 3.3824) -> (-2.75, 3.3824)
  line L512 (-2.75, 3.3824) -> (-2.75, -1.5)
  line L513 (-2.75, -1.5) -> (-3.25, -1.5)
  line L514 (-3.25, -1.5) -> (-3.25, 3.3824)
  line L515 (-3.25, 3.3824) -> (-2.75, -1.5) construction
  line L516 (-2.75, 3.3824) -> (-3.25, -1.5) construction
  line L517 (-2.25, 3.3824) -> (-1.75, 3.3824)
  line L518 (-1.75, 3.3824) -> (-1.75, -1.5)
  line L519 (-1.75, -1.5) -> (-2.25, -1.5)
  line L520 (-2.25, -1.5) -> (-2.25, 3.3824)
  line L521 (-2.25, 3.3824) -> (-1.75, -1.5) construction
  line L522 (-1.75, 3.3824) -> (-2.25, -1.5) construction
  line L523 (-1.25, 3.3824) -> (-0.75, 3.3824)
  line L524 (-0.75, 3.3824) -> (-0.75, -1.5)
  line L525 (-0.75, -1.5) -> (-1.25, -1.5)
  line L526 (-1.25, -1.5) -> (-1.25, 3.3824)
  line L527 (-1.25, 3.3824) -> (-0.75, -1.5) construction
  line L528 (-0.75, 3.3824) -> (-1.25, -1.5) construction
  line L529 (-0.25, 3.3824) -> (0.25, 3.3824)
  line L530 (0.25, 3.3824) -> (0.25, -1.5)
  line L531 (0.25, -1.5) -> (-0.25, -1.5)
  line L532 (-0.25, -1.5) -> (-0.25, 3.3824)
  line L533 (-0.25, 3.3824) -> (0.25, -1.5) construction
  line L534 (0.25, 3.3824) -> (-0.25, -1.5) construction
  line L535 (0.75, 3.3824) -> (1.25, 3.3824)
  line L536 (1.25, 3.3824) -> (1.25, -1.5)
  line L537 (1.25, -1.5) -> (0.75, -1.5)
  line L538 (0.75, -1.5) -> (0.75, 3.3824)
  line L539 (0.75, 3.3824) -> (1.25, -1.5) construction
  line L540 (1.25, 3.3824) -> (0.75, -1.5) construction
  line L541 (-9.25, 3.3824) -> (-8.75, 3.3824)
  line L542 (-8.75, 3.3824) -> (-8.75, -1.5)
  line L543 (-8.75, -1.5) -> (-9.25, -1.5)
  line L544 (-9.25, -1.5) -> (-9.25, 3.3824)
  line L545 (-9.25, 3.3824) -> (-8.75, -1.5) construction
  line L546 (-8.75, 3.3824) -> (-9.25, -1.5) construction
  line L547 (-8.25, 3.3824) -> (-7.75, 3.3824)
  line L548 (-7.75, 3.3824) -> (-7.75, -1.5)
  line L549 (-7.75, -1.5) -> (-8.25, -1.5)
  line L550 (-8.25, -1.5) -> (-8.25, 3.3824)
  line L551 (-8.25, 3.3824) -> (-7.75, -1.5) construction
  line L552 (-7.75, 3.3824) -> (-8.25, -1.5) construction
  line L553 (-7.25, 3.3824) -> (-6.75, 3.3824)
  line L554 (-6.75, 3.3824) -> (-6.75, -1.5)
  line L555 (-6.75, -1.5) -> (-7.25, -1.5)
  line L556 (-7.25, -1.5) -> (-7.25, 3.3824)
  line L557 (-7.25, 3.3824) -> (-6.75, -1.5) construction
  line L558 (-6.75, 3.3824) -> (-7.25, -1.5) construction
  line L559 (-6.25, 3.3824) -> (-5.75, 3.3824)
  line L560 (-5.75, 3.3824) -> (-5.75, -1.5)
  line L561 (-5.75, -1.5) -> (-6.25, -1.5)
  line L562 (-6.25, -1.5) -> (-6.25, 3.3824)
  line L563 (-6.25, 3.3824) -> (-5.75, -1.5) construction
  line L564 (-5.75, 3.3824) -> (-6.25, -1.5) construction
  line L565 (-5.25, 3.3824) -> (-4.75, 3.3824)
  line L566 (-4.75, 3.3824) -> (-4.75, -1.5)
  line L567 (-4.75, -1.5) -> (-5.25, -1.5)
  line L568 (-5.25, -1.5) -> (-5.25, 3.3824)
  line L569 (-5.25, 3.3824) -> (-4.75, -1.5) construction
  line L570 (-4.75, 3.3824) -> (-5.25, -1.5) construction
  line L571 (-4.25, 3.3824) -> (-3.75, 3.3824)
  line L572 (-3.75, 3.3824) -> (-3.75, -1.5)
  line L573 (-3.75, -1.5) -> (-4.25, -1.5)
  line L574 (-4.25, -1.5) -> (-4.25, 3.3824)
  line L575 (-4.25, 3.3824) -> (-3.75, -1.5) construction
  line L576 (-3.75, 3.3824) -> (-4.25, -1.5) construction
  line L577 (-3.25, 3.3824) -> (-2.75, 3.3824)
  line L578 (-2.75, 3.3824) -> (-2.75, -1.5)
  line L579 (-2.75, -1.5) -> (-3.25, -1.5)
  line L580 (-3.25, -1.5) -> (-3.25, 3.3824)
  line L581 (-3.25, 3.3824) -> (-2.75, -1.5) construction
  line L582 (-2.75, 3.3824) -> (-3.25, -1.5) construction
  line L583 (-2.25, 3.3824) -> (-1.75, 3.3824)
  line L584 (-1.75, 3.3824) -> (-1.75, -1.5)
  line L585 (-1.75, -1.5) -> (-2.25, -1.5)
  line L586 (-2.25, -1.5) -> (-2.25, 3.3824)
  line L587 (-2.25, 3.3824) -> (-1.75, -1.5) construction
  line L588 (-1.75, 3.3824) -> (-2.25, -1.5) construction
  line L589 (-1.25, 3.3824) -> (-0.75, 3.3824)
  line L590 (-0.75, 3.3824) -> (-0.75, -1.5)
  line L591 (-0.75, -1.5) -> (-1.25, -1.5)
  line L592 (-1.25, -1.5) -> (-1.25, 3.3824)
  line L593 (-1.25, 3.3824) -> (-0.75, -1.5) construction
  line L594 (-0.75, 3.3824) -> (-1.25, -1.5) construction
  line L595 (-0.25, 3.3824) -> (0.25, 3.3824)
  line L596 (0.25, 3.3824) -> (0.25, -1.5)
  line L597 (0.25, -1.5) -> (-0.25, -1.5)
  line L598 (-0.25, -1.5) -> (-0.25, 3.3824)
  line L599 (-0.25, 3.3824) -> (0.25, -1.5) construction
  line L600 (0.25, 3.3824) -> (-0.25, -1.5) construction
  point P0 (0, 0)
  point P1 (0, 0.9412)
  point P2 (1, 0.9412)
  point P3 (2, 0.9412)
  point P4 (3, 0.9412)
  point P5 (4, 0.9412)
  point P6 (5, 0.9412)
  point P7 (6, 0.9412)
  point P8 (7, 0.9412)
  point P9 (8, 0.9412)
  point P10 (9, 0.9412)
  point P11 (-1, 0.9412)
  point P12 (0, 0.9412)
  point P13 (1, 0.9412)
  point P14 (2, 0.9412)
  point P15 (3, 0.9412)
  point P16 (4, 0.9412)
  point P17 (5, 0.9412)
  point P18 (6, 0.9412)
  point P19 (7, 0.9412)
  point P20 (8, 0.9412)
  point P21 (-2, 0.9412)
  point P22 (-1, 0.9412)
  point P23 (0, 0.9412)
  point P24 (1, 0.9412)
  point P25 (2, 0.9412)
  point P26 (3, 0.9412)
  point P27 (4, 0.9412)
  point P28 (5, 0.9412)
  point P29 (6, 0.9412)
  point P30 (7, 0.9412)
  point P31 (-3, 0.9412)
  point P32 (-2, 0.9412)
  point P33 (-1, 0.9412)
  point P34 (0, 0.9412)
  point P35 (1, 0.9412)
  point P36 (2, 0.9412)
  point P37 (3, 0.9412)
  point P38 (4, 0.9412)
  point P39 (5, 0.9412)
  point P40 (6, 0.9412)
  point P41 (-4, 0.9412)
  point P42 (-3, 0.9412)
  point P43 (-2, 0.9412)
  point P44 (-1, 0.9412)
  point P45 (0, 0.9412)
  point P46 (1, 0.9412)
  point P47 (2, 0.9412)
  point P48 (3, 0.9412)
  point P49 (4, 0.9412)
  point P50 (5, 0.9412)
  point P51 (-5, 0.9412)
  point P52 (-4, 0.9412)
  point P53 (-3, 0.9412)
  point P54 (-2, 0.9412)
  point P55 (-1, 0.9412)
  point P56 (0, 0.9412)
  point P57 (1, 0.9412)
  point P58 (2, 0.9412)
  point P59 (3, 0.9412)
  point P60 (4, 0.9412)
  point P61 (-6, 0.9412)
  point P62 (-5, 0.9412)
  point P63 (-4, 0.9412)
  point P64 (-3, 0.9412)
  point P65 (-2, 0.9412)
  point P66 (-1, 0.9412)
  point P67 (0, 0.9412)
  point P68 (1, 0.9412)
  point P69 (2, 0.9412)
  point P70 (3, 0.9412)
  point P71 (-7, 0.9412)
  point P72 (-6, 0.9412)
  point P73 (-5, 0.9412)
  point P74 (-4, 0.9412)
  point P75 (-3, 0.9412)
  point P76 (-2, 0.9412)
  point P77 (-1, 0.9412)
  point P78 (0, 0.9412)
  point P79 (1, 0.9412)
  point P80 (2, 0.9412)
  point P81 (-8, 0.9412)
  point P82 (-7, 0.9412)
  point P83 (-6, 0.9412)
  point P84 (-5, 0.9412)
  point P85 (-4, 0.9412)
  point P86 (-3, 0.9412)
  point P87 (-2, 0.9412)
  point P88 (-1, 0.9412)
  point P89 (0, 0.9412)
  point P90 (1, 0.9412)
  point P91 (-9, 0.9412)
  point P92 (-8, 0.9412)
  point P93 (-7, 0.9412)
  point P94 (-6, 0.9412)
  point P95 (-5, 0.9412)
  point P96 (-4, 0.9412)
  point P97 (-3, 0.9412)
  point P98 (-2, 0.9412)
  point P99 (-1, 0.9412)
  point P100 (0, 0.9412)
  dimension "d4" = 0.5
  dimension "d5" = 1
  dimension "d8" = 1
  dimension "d11" = 1
  constraints: 1200 end point, 3 horizontal, 2 midpoint, 2 parallel, 1 perpendicular, 1 vertical alignment, 1089 other
  measures "d4" distance of L0.start L0.end
  measures "d5" distance between parallel lines of L6 L2
  measures "d8" distance of L0.start L7.start
  measures "d11" distance of L0.start L61.start
extrude "Extrusion2" cut sketch "Sketch2" against normal blind 20
body "Solid1"
